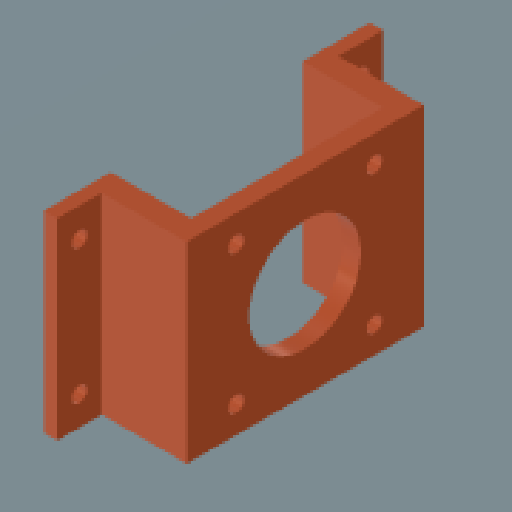
# Autodesk Inventor part: Z Axis Motor Bracket
Saved by Autodesk Inventor 2023.2 (Build 272271000, 271)
## iProperties
Created: 2023-02-19
Part Number: Z Axis Motor Bracket
Material: ABS Plastic
Document SubType Name: Modeling
Designer: remop
Density: 1.06 g/cm^3
Appearance: Smooth - Light Orange
Author: remop
Autodesk Inventor part; units mm, degrees
ref_plane "YZ Plane" through (0, 0, 0) normal (1, 0, 0) x (0, 1, 0)
ref_plane "XZ Plane" through (0, 0, 0) normal (0, 1, 0) x (-1, 0, 0)
ref_plane "XY Plane" through (0, 0, 0) normal (0, 0, 1) x (1, 0, 0)
sketch "Sketch1" plane through (0, 0, 0) normal (1, 0, 0) x (0, 1, 0)
  circle A0 centre (0, 0) radius 12.5
  circle A1 centre (-15.5, -15.5) radius 1.75
  circle A2 centre (15.5, -15.5) radius 1.75
  circle A3 centre (15.5, 15.5) radius 1.75
  circle A4 centre (-15.5, 15.5) radius 1.75
  line L0 (21.5, -21.5) -> (-21.5, -21.5)
  line L1 (-21.5, -21.5) -> (-21.5, 21.5)
  line L2 (-21.5, 21.5) -> (21.5, 21.5)
  line L3 (21.5, 21.5) -> (21.5, -21.5)
  line L4 (21.5, -21.5) -> (-21.5, 21.5) construction
  line L5 (-21.5, -21.5) -> (21.5, 21.5) construction
  dimension "d2" = 360
  dimension "d4" = 3.5
  dimension "d5" = 25
  dimension "d6" = 31
  dimension "d7" = 43
  constraints: 12 end point, 5 centre point, 2 midpoint, 2 parallel, 2 perpendicular, 1 coincident, 1 horizontal, 1 vertical alignment, 9 other
  measures "d4" diameter of A4
  measures "d5" diameter of A0
  measures "d6" distance of A1.centre A4.centre
  measures "d7" distance of L0.end L1.end
extrude "Extrusion1" add sketch "Sketch1" along normal blind 4
sketch "Sketch5" plane through (0, 21.5, 21.5) normal (0, 1, 0) x (1, 0, 0)
  line L0 (0, 43) -> (0, 0) projected
  line L1 (0, 0) -> (4, 0) projected
  line L2 (4, 43) -> (4, 0) projected
  line L3 (0, 43) -> (4, 43) projected
  line L4 (0, 43) -> (4, 43) projected
  line L5 (0, 43) -> (-18, 43)
  line L6 (-18, 43) -> (-18, 58)
  line L7 (-18, 58) -> (-15, 58)
  line L8 (-15, 58) -> (-15, 48)
  line L9 (-15, 48) -> (4, 48)
  line L10 (4, 48) -> (4, 43)
  line L11 (0, 0) -> (-18, 0)
  line L12 (-18, 0) -> (-18, -15)
  line L13 (-18, -15) -> (-15, -15)
  line L14 (-15, -15) -> (-15, -5)
  line L15 (-15, -5) -> (4, -5)
  line L16 (4, -5) -> (4, 0)
  line L17 (4, 43) -> (4, 0) projected
  point P0 (0, 21.5)
  dimension "d17" = 5
  dimension "d18" = 3
  dimension "d19" = 10
  dimension "d23" = 22
  constraints: 24 end point, 9 perpendicular, 4 equal length, 2 horizontal, 1 point on line, 1 vertical, 1 vertical alignment
  measures "d17" distance between parallel lines of L5 L9
  measures "d18" distance between parallel lines of L6 L8
  measures "d19" distance of L7.end L8.end
  measures "d23" distance between parallel lines of L2 L12
extrude "Extrusion4" add sketch "Sketch5" against normal up to surface (43 mm away) contours L5 L6 L7 L8 L9 L10 L3 | L1 L16 L15 L14 L13 L12 L11
sketch "Sketch6" plane through (-15, 21.5, 36.5) normal (1, 0, 0) x (0, 0, -1)
  line L0 (0, -43) -> (10, -43) projected
  line L1 (10, 0) -> (10, -43) projected
  line L2 (0, 0) -> (10, 0) projected
  line L3 (0, 0) -> (0, -43) projected
  line L4 (63, -43) -> (73, -43) projected
  line L5 (73, 0) -> (73, -43) projected
  line L6 (63, 0) -> (73, 0) projected
  line L7 (63, 0) -> (63, -43) projected
  point P0 (36.5, -21.5)
  point P1 (5, -6.5)
  point P2 (5, -36.5)
  point P3 (68, -36.5)
  point P4 (68, -6.5)
  point P5 (5, 0)
  point P6 (5, -43)
  point P7 (68, -43)
  point P8 (68, 0)
  dimension "d24" = 6.5
  dimension "d25" = 6.5
  dimension "d26" = 30
  constraints: 4 midpoint, 4 vertical alignment, 2 horizontal alignment
  measures "d24" distance from line of L2 point (5, -6.5)
  measures "d25" distance from line of L0 point (5, -36.5)
  measures "d26" distance of point (5, -36.5) point (5, -6.5)
hole "Hole1" at (-15, 15, 31.5) at (-15, -15, 31.5) at (-15, -15, -31.5) at (-15, 15, -31.5) direction (-1, 0, 0) diameter 3.5 end through all
equation "\"d25\" = d24"
body "Solid1"
